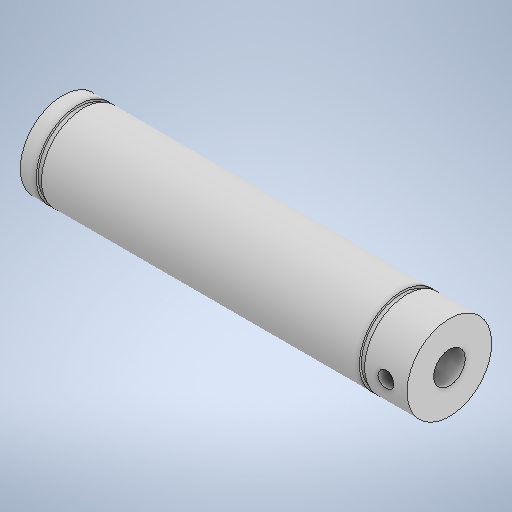
# Autodesk Inventor part: shaft potmeter
Saved by Autodesk Inventor 2025.2 (Build 292293000, 293)
## iProperties
Created: 2025-05-13
Part Number: shaft potmeter
Material: Generic
Document SubType Name: Modeling
Designer: Caspe
Density: 1 g/cm^3
Appearance: Default
Author: Caspe
Autodesk Inventor part; units mm, degrees
ref_plane "YZ Plane" through (0, 0, 0) normal (1, 0, 0) x (0, 1, 0)
ref_plane "XZ Plane" through (0, 0, 0) normal (0, 1, 0) x (-1, 0, 0)
ref_plane "XY Plane" through (0, 0, 0) normal (0, 0, 1) x (1, 0, 0)
sketch "Sketch1" plane through (0, 0, 0) normal (0, 0, 1) x (1, 0, 0)
  line L0 (0, 0) -> (73, 0)
  line L1 (73, 0) -> (73, 8)
  line L2 (73, 8) -> (0, 8)
  line L3 (0, 8) -> (0, 0)
  line L4 (64, 8) -> (65, 8)
  line L5 (65, 8) -> (65, 7.6)
  line L6 (65, 7.6) -> (64, 7.6)
  line L7 (64, 7.6) -> (64, 8)
  line L8 (36.5, 8) -> (36.5, 0)
  line L9 (73, 0) -> (58, 0)
  line L10 (58, 0) -> (58, 3)
  line L11 (58, 3) -> (73, 3)
  line L12 (73, 3) -> (73, 0)
  line L13 (3, 8) -> (4, 8)
  line L14 (4, 8) -> (4, 7.6)
  line L15 (4, 7.6) -> (3, 7.6)
  line L16 (3, 7.6) -> (3, 8)
  point P0 (64.5, 7.6)
  point P1 (65, 7.8)
  point P2 (58, 0)
  point P3 (73, 3)
  point P4 (65, 8)
  dimension "d0" = 73
  dimension "d1" = 8
  dimension "d2" = 1
  dimension "d3" = 7.6
  dimension "d4" = 8
  dimension "d5" = 15
  dimension "d6" = 3
  dimension "d8" = 1
  dimension "d9" = 7.6
  dimension "d10" = 3
  constraints: 34 end point, 8 parallel, 4 horizontal, 4 midpoint, 4 perpendicular, 2 point on line
  measures "d0" distance of L2.end L1.end
  measures "d1" distance of L1.end L0.end
  measures "d2" distance of L5.end L6.end
  measures "d3" distance from line of point (64.5, 7.6) L0
  measures "d4" distance from line of L1 point (65, 7.8)
  measures "d5" distance of L10.end L11.end
  measures "d6" distance of L9.end L10.end
  measures "d8" distance between parallel lines of L14 L16
  measures "d9" distance between parallel lines of L0 L15
  measures "d10" distance between parallel lines of L3 L16
revolve "Revolution1" add sketch "Sketch1" angle 360 about axis through (0, 0, 0) along (1, 0, 0) contours L3 L2 L16 L15 L14 L8 L0 | L8 L2 L7 L6 L5 L1 L11 L10 L0
sketch "Sketch2" plane through (0, 0, 0) normal (0, 0, 1) x (1, 0, 0)
  line L0 (73, -3) -> (73, 3) projected
  line L1 (58, -3) -> (58, 3) projected
  circle A0 centre (69, 0) radius 1.5
  point P0 (0, 0)
  dimension "d11" = 3
  dimension "d12" = 4
  constraints: 1 centre point
  measures "d11" diameter of A0
  measures "d12" distance from line of L0 A0.centre
extrude "Extrusion1" cut sketch "Sketch2" along normal blind 10
body "Solid1"
